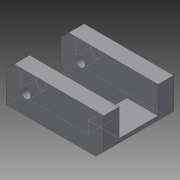
# Autodesk Inventor part: Top pully rack
Saved by Autodesk Inventor 2015 (Build 190159000, 159)
## iProperties
Created: 2019-01-17
Part Number: Top pully rack
Material: Generic
Document SubType Name: Modeling
Designer: Toby
Density: 1 g/cm^3
Appearance: Default
Author: Toby
Autodesk Inventor part; units mm, degrees
ref_plane "YZ Plane" through (0, 0, 0) normal (1, 0, 0) x (0, 1, 0)
ref_plane "XZ Plane" through (0, 0, 0) normal (0, 1, 0) x (-1, 0, 0)
ref_plane "XY Plane" through (0, 0, 0) normal (0, 0, 1) x (1, 0, 0)
sketch "Sketch1" plane through (0, 0, 0) normal (0, 0, 1) x (1, 0, 0)
  line L0 (-23.4386, 9.1579) -> (1.5614, 9.1579)
  line L1 (1.5614, 9.1579) -> (1.5614, 5.1579)
  line L2 (1.5614, 5.1579) -> (-23.4386, 5.1579)
  line L3 (-23.4386, 5.1579) -> (-23.4386, 9.1579)
  line L4 (-23.4386, -4.8421) -> (1.5614, -4.8421)
  line L5 (1.5614, -4.8421) -> (1.5614, -8.8421)
  line L6 (1.5614, -8.8421) -> (-23.4386, -8.8421)
  line L7 (-23.4386, -8.8421) -> (-23.4386, -4.8421)
  point P0 (0, 0)
  dimension "d0" = 4
  dimension "d1" = 4
  dimension "d2" = 10
  dimension "d3" = 25
  dimension "d4" = 25
  constraints: 16 end point, 4 parallel, 2 horizontal, 2 perpendicular, 1 collinear
  measures "d0" distance between parallel lines of L2 L0
  measures "d1" distance between parallel lines of L6 L4
  measures "d2" distance between parallel lines of L4 L2
  measures "d3" distance between parallel lines of L1 L3
  measures "d4" distance between parallel lines of L7 L5
extrude "Extrusion1" add sketch "Sketch1" along normal blind 10
sketch "Sketch2" plane through (0, 0, 0) normal (0, 0, -1) x (-1, 0, 0)
  line L0 (-1.5614, -8.8421) -> (6.4386, -8.8421)
  line L1 (6.4386, -8.8421) -> (6.4386, 9.1579)
  line L2 (6.4386, 9.1579) -> (-1.5614, 9.1579)
  line L3 (-1.5614, 9.1579) -> (-1.5614, -8.8421)
  line L4 (23.4386, 9.1579) -> (-1.5614, 9.1579) projected
  point P0 (0, 0)
  dimension "d7" = 8
  constraints: 8 end point, 2 parallel, 1 collinear, 1 horizontal, 1 perpendicular
  measures "d7" distance between parallel lines of L1 L3
extrude "Extrusion2" add sketch "Sketch2" against normal blind 3
sketch "Sketch3" plane through (-23.4386, -8.8421, 0) normal (0, -1, 0) x (1, 0, 0)
  line L0 (0, 0) -> (0, 10) projected
  circle A0 centre (5, 5) radius 1.25
  point P0 (23.4386, 0)
  dimension "d10" = 5
  dimension "d11" = 2.5
  constraints: 1 centre point, 1 coincident
  measures "d10" distance from line of L0 point (5, 5)
  measures "d11" diameter of A0
extrude "Extrusion3" cut sketch "Sketch3" against normal blind 30
chamfer "Chamfer1" distance 2 angle 45 1 edges at (1.5614, 0.1579, 0)
chamfer "Chamfer2" distance 2 angle 45 2 edges at (-23.4386, 7.1579, 10) (-23.4386, -6.8421, 10)
body "Solid1"
